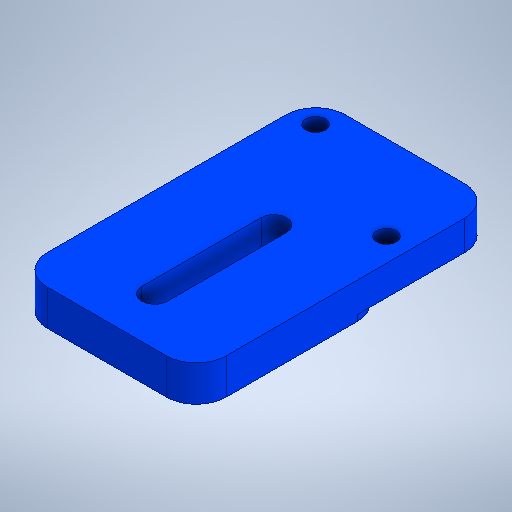
# Autodesk Inventor part: LimitSwitch
Saved by Autodesk Inventor 2025.2 (Build 292293000, 293)
## iProperties
Created: 2025-09-16
Part Number: LimitSwitch
Material: Generic
Document SubType Name: Modeling
Designer: Simon
Density: 1 g/cm^3
Appearance: Default(1)
Author: Simon
Autodesk Inventor part; units mm, degrees
ref_plane "YZ Plane" through (0, 0, 0) normal (1, 0, 0) x (0, 1, 0)
ref_plane "XZ Plane" through (0, 0, 0) normal (0, 1, 0) x (-1, 0, 0)
ref_plane "XY Plane" through (0, 0, 0) normal (0, 0, 1) x (1, 0, 0)
sketch "Sketch1" plane through (0, 0, 0) normal (0, 1, 0) x (-1, 0, 0)
  line L0 (0, 0) -> (30, 0)
  line L1 (30, 0) -> (30, -50)
  line L2 (30, -50) -> (0, -50)
  line L3 (0, -50) -> (0, 0)
  dimension "d0" = 30
  dimension "d1" = 50
  constraints: 8 end point, 2 parallel, 1 horizontal, 1 perpendicular
  measures "d0" distance of L1.end L2.end
  measures "d1" distance of L0.end L1.end
extrude "Extrusion1" add sketch "Sketch1" along normal blind 5
fillet "Fillet1" radius 5 4 edges at (-30, 2.5, 0) (0, 2.5, 0) (0, 2.5, -50) (-30, 2.5, -50)
sketch "Sketch2" plane through (0, 5, 0) normal (0, 1, 0) x (1, 0, 0)
  line L0 (-5, 50) -> (-25, 50) projected
  line L1 (-15, 50) -> (-15, 46.1)
  line L2 (-15, 46.1) -> (-26.1, 46.1)
  line L3 (-26.1, 46.1) -> (-3.9, 46.1)
  line L4 (-3.9, 46.1) -> (-3.9, 35.8)
  circle A0 centre (-26.1, 46.1) radius 1.65
  circle A1 centre (-3.9, 35.8) radius 1.65
  line L5 (-25, 0) -> (-5, 0) projected
  line L6 (-15, 0) -> (-15, 50)
  line L7 (-15, 0) -> (-15, 8)
  circle A2 centre (-15, 8) radius 2.15
  line L8 (-15, 8) -> (-15, 28)
  circle A3 centre (-15, 28) radius 2.15
  line L9 (-17.15, 8) -> (-17.15, 28)
  line L10 (-12.85, 28) -> (-12.85, 8)
  point P0 (0, 0)
  dimension "d5" = 3.9
  dimension "d6" = 11.1
  dimension "d7" = 22.2
  dimension "d8" = 10.3
  dimension "d9" = 3.3
  dimension "d10" = 3.3
  dimension "d11" = 8
  dimension "d12" = 4.3
  dimension "d13" = 20
  dimension "d14" = 4.3
  constraints: 18 end point, 4 centre point, 4 coincident, 4 point on circle, 3 point on line, 2 midpoint, 2 perpendicular, 2 tangent, 1 collinear, 1 vertical
  measures "d5" distance of L1.start L1.end
  measures "d6" distance of L1.end L2.end
  measures "d7" distance of L2.end L3.end
  measures "d8" distance of L3.end L4.end
  measures "d9" diameter of A0
  measures "d10" diameter of A1
  measures "d11" distance of L6.start L7.end
  measures "d12" diameter of A2
  measures "d13" distance of L8.start L8.end
  measures "d14" diameter of A3
sketch "Sketch3" plane through (0, 0, 0) normal (0, -1, 0) x (1, 0, 0)
  line L0 (-30, -45) -> (-30, -5) projected
  line L1 (0, 0) -> (-30, 0)
  line L2 (-30, 0) -> (-30, -32)
  line L3 (-30, -32) -> (0, -32)
  line L4 (0, -32) -> (0, 0)
  dimension "d15" = 32
  constraints: 8 end point, 2 parallel, 1 horizontal, 1 perpendicular, 1 point on line
  measures "d15" distance of L2.end L1.end
extrude "Extrusion2" add sketch "Sketch3" along normal blind 1
fillet "Fillet2" radius 5 4 edges at (0, -0.5, 0) (0, -0.5, -32) (-30, -0.5, 0) (-30, -0.5, -32)
extrude "Extrusion3" cut sketch "Sketch2" against normal through all
body "Solid1"
